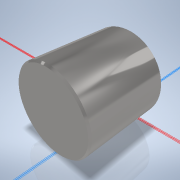
# Autodesk Inventor part: ciezarek
Saved by Autodesk Inventor 2021 (Build 250183000, 183)
## iProperties
Created: 2021-11-16
Part Number: ciezarek
Material: Stal nierdzewna 440C
Document SubType Name: Modeling
Designer: wojwo
Mass: 49.9978 g
Surface Area: 19.0242 cm^2
Volume: 6.45133 cm^3
Density: 7.75 g/cm^3
Appearance: Częściowo polerowana
Author: wojwo
Autodesk Inventor part; units mm, degrees
ref_plane "YZ Plane" through (0, 0, 0) normal (1, 0, 0) x (0, 1, 0)
ref_plane "XZ Plane" through (0, 0, 0) normal (0, 1, 0) x (-1, 0, 0)
ref_plane "XY Plane" through (0, 0, 0) normal (0, 0, 1) x (1, 0, 0)
sketch "Szkic1" plane through (0, 0, 0) normal (0, 0, 1) x (1, 0, 0)
  circle A0 centre (0, -7.5) radius 4.5 projected
  circle A1 centre (0, 0) radius 39.6 projected
  circle A2 centre (0, 7.5) radius 4.5 projected
  circle A3 centre (0, -7.5) radius 4.5 projected
  circle A4 centre (0, 0) radius 39.6 projected
  circle A5 centre (0, 7.5) radius 4.5 projected
  circle A6 centre (0, 25) radius 11
  point P0 (0, 0)
  dimension "d0" = 22
  dimension "d6" = 25
  constraints: 1 centre point
  measures "d0" diameter of A6
  measures "d6" distance of point (0, 0) A6.centre
extrude "Wyciągnięcie proste1" add sketch "Szkic1" along normal blind 17 contours A6
chamfer "Faza1" distance 0.4 angle 45 2 edges at (-11, 25, 0) (-11, 25, 17)
